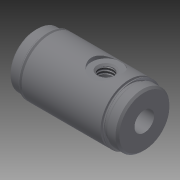
# Autodesk Inventor part: D-68355---0
Saved by Autodesk Inventor 2014 (Build 180170000, 170)
## iProperties
Category: PARTsolutions
Company: BIMBA
Created: 2014-01-19
Part Number: D-68355---0
Material: Generic
Catalog Web Link: www.cadenas.de
Description: Center Section Cyl-Original Line Cyl
Vendor: BIMBA
Document SubType Name: Standard Catalog Part
Designer: Michael
Manufacturer: BIMBA
Density: 1 g/cm^3
Appearance: RGB(211.00000262260440,211.00000262260440,211.00000262260440)
PSOL_IDENT_0: {$CADENAS_DATA\23d-libs\bimba\bimba\bimba_imperial\bimba_full_line\original_line_cylinders\three_pos
PSOL_IDENT_1: ition_cylinders\center_section_cyl.prj},192 {VTYP=3D},{NB=D-68355---0},{LINA=D-68355---0},{NN=Center
PSOL_IDENT_2: Section Cyl},{DATE=05.12.2012 11:45:13},{GEOMDATE=05.12.2012 10:10:00},{VERSION=},{LINEID=10},{LINE
PSOL_IDENT_3: SUBID=-1},{WBVAR=MNT,BUMPER,STRED}  {NB=D-68355---0},{LINA=D-68355---0},{KT=DUMMY},{PN=D-68355},{MNT=
PSOL_IDENT_4: },{BUMPER=},{DRAW=1},{DRAWC=1},{DRAWC1=1},{A=1.15600000},{A1=0.40600000},{A2=0.18800000},{A3=0.31460
PSOL_IDENT_5: 000},{A4=0.15860000},{A5=0.00000000},{A6=0.50000000},{A66=0.00000000},{A7=0.13200000},{A8=0.02500000
PSOL_IDENT_6: },{A9=0.00000000},{A10=0.84},{A11=0.00000000},{A12=0.02500000},{A13=0.132},{B=0.61500000},{B1=0.0000
PSOL_IDENT_7: 0000},{B2=0.57300000},{B3=0.52300000},{C=0.37500000},{C1=0.25050000},{C11=0.17320000},{C2=0.31950000
PSOL_IDENT_8: },{C3=0.00000000},{C4=0.34400000},{C44=0.00000000},{CH=0.02000000},{CH1=0.02500000},{CH2=0.01000000}
PSOL_IDENT_9: ,{ND=UNF},{D=0.19000000},{DCH=0.03000000},{D11=0.31200000},{D11DP=0.04000000},{A1B=0.00000000},{A1P=
PSOL_IDENT_10: 1.15600000},{A1N=1.03100000},{A4P=0.15700000},{A4N=0.53100000},{A55=0.02500000},{GG=0},{A111=1.156},
PSOL_IDENT_11: {A44=0.157},{ID=0.5725},{OD=0.615},{D1=0.61500000},{D2=0.57250000},{RP=0.02185660},{ADD1=0.00200000}
PSOL_IDENT_12: ,{ADD2=0.00200000},{ADD11=0.00000000},{ADD22=0.00400000},{ADDER=0.133},{AA10=0.84000000},{AA11=0.842
PSOL_IDENT_13: 00000},{D5=0.19000000},{STRED=0.00000}
CNS_NN: Center Section Cyl
CNS_NT: Original Line Cyl
CNS_NB: D-68355---0
CNS_NBSYN: $PN.-$MNT.-$BUMPER.-$STRED.
CNS_LINA: D-68355---0
CNS_PN: D-68355
CNS_MNT: Nose Mounting
CNS_BUMPER: w/o Bumper
CNS_DRAW: 1
CNS_DRAWC: 1
CNS_DRAWC1: 1
CNS_A: 1.15600000
CNS_A1: 0.40600000
CNS_A2: 0.18800000
CNS_A3: 0.31460000
CNS_A4: 0.15860000
CNS_A5: 0.00000000
CNS_A6: 0.50000000
CNS_A66: 0.00000000
CNS_A7: 0.13200000
CNS_A8: 0.02500000
CNS_A9: 0.00000000
CNS_A10: 0.840
CNS_A11: 0.00000000
CNS_A12: 0.02500000
CNS_A13: 0.132
CNS_B: 0.61500000
CNS_B1: 0.00000000
CNS_B2: 0.57300000
CNS_B3: 0.52300000
CNS_C: 0.37500000
CNS_C1: 0.25050000
CNS_C11: 0.17320000
CNS_C2: 0.31950000
CNS_C3: 0.00000000
CNS_C4: 0.34400000
CNS_C44: 0.00000000
CNS_CH: 0.02000000
CNS_CH1: 0.02500000
CNS_CH2: 0.01000000
CNS_ND: UNF
CNS_D: 0.19000000
CNS_DCH: 0.03000000
CNS_D11: 0.31200000
CNS_D11DP: 0.04000000
CNS_A1B: 0.00000000
CNS_A1P: 1.15600000
CNS_A1N: 1.03100000
CNS_A4P: 0.15700000
CNS_A4N: 0.53100000
CNS_A55: 0.02500000
CNS_GG: 0.000
CNS_A111: 1.156
CNS_A44: 0.157
CNS_ID: 0.573
CNS_OD: 0.615
CNS_D1: 0.61500000
CNS_D2: 0.57250000
CNS_RP: 0.02185660
CNS_ADD1: 0.00200000
CNS_ADD2: 0.00200000
CNS_ADD11: 0.00000000
CNS_ADD22: 0.00400000
CNS_ADDER: 0.133
CNS_AA10: 0.84000000
CNS_AA11: 0.84200000
CNS_D5: 0.19000000
CNS_STRED: 0.00000
SUPPLIER: BIMBA
ARTICLENO: D-68355---0
BOMINFO: D-68355---0
CREATOR: CADENAS GmbH
Title: D-68355---0
Author: Cadenas PARTsolutions
Comments: Original Line Cyl
Autodesk Inventor part; units mm, degrees
sketch "Sketch_1" plane through (0, 0, 0) normal (0, 0, 1) x (1, 0, 0)
  line L0 (29.3624, 0) -> (0, 0)
  line L1 (0, 0) -> (0, 6.7691)
  line L2 (0, 6.7691) -> (0.508, 7.2771)
  line L3 (0.508, 7.2771) -> (2.7432, 7.2771)
  line L4 (2.7432, 7.2771) -> (3.3782, 6.6421)
  line L5 (3.3782, 6.6421) -> (4.0132, 6.6421)
  line L6 (4.0132, 6.6421) -> (4.0132, 7.8105)
  line L7 (4.0132, 7.8105) -> (25.3492, 7.8105)
  line L8 (25.3492, 7.8105) -> (25.3492, 6.6421)
  line L9 (25.3492, 6.6421) -> (25.9842, 6.6421)
  line L10 (25.9842, 6.6421) -> (26.6192, 7.2771)
  line L11 (26.6192, 7.2771) -> (28.8544, 7.2771)
  line L12 (28.8544, 7.2771) -> (29.3624, 6.7691)
  line L13 (29.3624, 6.7691) -> (29.3624, 0)
  line L14 (29.3624, 0) -> (0, 0)
  constraints: 30 end point
revolve "Revolution1" add sketch "Sketch_1" angle 360 about axis through (29.3624, 0, 0) along (1, 0, 0)
sketch "Sketch2" plane through (29.3624, 0, 0) normal (1, 0, 0) x (0, 0, -1)
  point P0 (0, 0)
hole "Hole1" at (29.3624, 0, 0) direction (-1, 0, 0) diameter 5.334 depth 29.3624
sketch "Sketch_6" plane through (0, 0, 0) normal (0, 0, 1) x (1, 0, 0)
  line L0 (19.05, 0) -> (19.05, 7.8105)
  line L1 (19.05, 7.8105) -> (23.0124, 7.8105)
  line L2 (23.0124, 7.8105) -> (23.0124, 6.7945)
  line L3 (23.0124, 6.7945) -> (21.463, 6.7945)
  line L4 (21.463, 6.7945) -> (21.0337, 6.3652)
  line L5 (21.0337, 6.3652) -> (21.0337, 0)
  line L6 (21.0337, 0) -> (19.05, 0)
  line L7 (19.05, 0) -> (19.05, 7.8105)
  constraints: 16 end point
revolve "Revolution2" cut sketch "Sketch_6" angle 360 about axis through (19.05, 0, 0) along (0, -1, 0)
thread "Thread1" size "10-32 UNF" class "2B" standard "ANSI Unified Screw Threads" length 2.4257 offset 2.5862
sketch "Sketch_8" plane through (0, 0, 0) normal (0, 0, 1) x (1, 0, 0)
  line L0 (29.3624, 0) -> (-29.3624, 0)
  line L1 (24.7988, 6.6421) -> (25.0862, 6.6421)
  line L2 (25.0862, 6.6421) -> (26.1874, 7.7433)
  line L3 (26.1874, 7.7433) -> (26.1874, 7.8105)
  line L4 (26.1874, 7.8105) -> (25.9672, 7.8105)
  line L5 (25.9672, 7.8105) -> (24.7988, 6.6421)
  constraints: 12 end point
revolve "Revolution3" add sketch "Sketch_8" angle 360 about axis through (29.3624, 0, 0) along (1, 0, 0)
sketch "Sketch_14" plane through (0, 0, 0) normal (0, 0, 1) x (1, 0, 0)
  line L0 (29.3624, 0) -> (-29.3624, 0)
  line L1 (3.175, 7.7433) -> (4.2762, 6.6421)
  line L2 (4.2762, 6.6421) -> (4.5636, 6.6421)
  line L3 (4.5636, 6.6421) -> (3.3952, 7.8105)
  line L4 (3.3952, 7.8105) -> (3.175, 7.8105)
  line L5 (3.175, 7.8105) -> (3.175, 7.7433)
  constraints: 12 end point
revolve "Revolution4" add sketch "Sketch_14" angle 360 about axis through (29.3624, 0, 0) along (1, 0, 0)
ref_plane "ba2_XY" through (19.05, 7.8105, 0) normal (0, 0, 1) x (1, 0, 0)
ref_plane "ba2_YZ" through (19.05, 7.8105, 0) normal (1, 0, 0) x (0, 1, 0)
ref_plane "ba2_ZX" through (19.05, 7.8105, 0) normal (0, 1, 0) x (0, 0, 1)
ref_plane "centar_XY" through (14.6812, 0, 0) normal (1, 0, 0) x (0, 0, -1)
ref_plane "centar_YZ" through (14.6812, 0, 0) normal (0, 0, -1) x (0, 1, 0)
ref_plane "centar_ZX" through (14.6812, 0, 0) normal (0, 1, 0) x (1, 0, 0)
ref_plane "d1_XY" through (21.463, 6.7945, 0) normal (0, 0, 1) x (1, 0, 0)
ref_plane "d1_YZ" through (21.463, 6.7945, 0) normal (1, 0, 0) x (0, 1, 0)
ref_plane "d1_ZX" through (21.463, 6.7945, 0) normal (0, 1, 0) x (0, 0, 1)
ref_plane "d2_XY" through (16.637, 6.7945, 0) normal (0, 0, 1) x (1, 0, 0)
ref_plane "d2_YZ" through (16.637, 6.7945, 0) normal (1, 0, 0) x (0, 1, 0)
ref_plane "d2_ZX" through (16.637, 6.7945, 0) normal (0, 1, 0) x (0, 0, 1)
ref_plane "to_cyl_A_XY" through (2.7432, 0, 0) normal (1, 0, 0) x (0, 0, -1)
ref_plane "to_cyl_A_YZ" through (2.7432, 0, 0) normal (0, 0, -1) x (0, 1, 0)
ref_plane "to_cyl_A_ZX" through (2.7432, 0, 0) normal (0, 1, 0) x (1, 0, 0)
ref_plane "to_cyl_B_XY" through (26.6192, 0, 0) normal (1, 0, 0) x (0, 0, -1)
ref_plane "to_cyl_B_YZ" through (26.6192, 0, 0) normal (0, 0, -1) x (0, 1, 0)
ref_plane "to_cyl_B_ZX" through (26.6192, 0, 0) normal (0, 1, 0) x (1, 0, 0)
ref_plane "to_rod_A_XY" through (29.3624, 0, 0) normal (1, 0, 0) x (0, 0, -1)
ref_plane "to_rod_A_YZ" through (29.3624, 0, 0) normal (0, 0, -1) x (0, 1, 0)
ref_plane "to_rod_A_ZX" through (29.3624, 0, 0) normal (0, 1, 0) x (1, 0, 0)
body "Solid1"
